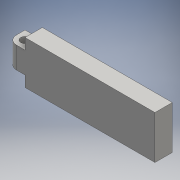
# Autodesk Inventor part: promo3
Saved by Autodesk Inventor 2016 (Build 200138000, 138)
## iProperties
Created: 2016-05-09
Part Number: promo3
Material: 一般
Document SubType Name: Modeling
Designer: 宏太
Density: 1 g/cm^3
Appearance: 既定
Author: 宏太
Autodesk Inventor part; units mm, degrees
ref_plane "YZ Plane" through (0, 0, 0) normal (1, 0, 0) x (0, 1, 0)
ref_plane "XZ Plane" through (0, 0, 0) normal (0, 1, 0) x (-1, 0, 0)
ref_plane "XY Plane" through (0, 0, 0) normal (0, 0, 1) x (1, 0, 0)
sketch "スケッチ1" plane through (0, 0, 0) normal (0, 1, 0) x (-1, 0, 0)
  line L0 (0, 0) -> (30, 0)
  line L1 (30, 10) -> (0, 10)
  line L2 (0, 10) -> (0, 0)
  line L3 (30, 7.5) -> (34, 7.5)
  line L4 (34, 7.5) -> (34, 2.5)
  line L5 (34, 2.5) -> (30, 2.5)
  line L6 (30, 10) -> (30, 7.5)
  line L7 (30, 2.5) -> (30, 0)
  dimension "d0" = 30
  dimension "d1" = 10
  dimension "d5" = 5
  dimension "d6" = 2.5
  constraints: 16 end point, 2 equal length, 2 horizontal, 1 perpendicular, 1 vertical
  measures "d0" distance of L1.end L1.start
  measures "d1" distance of L1.start L0.end
  measures "d5" distance between parallel lines of L3 L5
  measures "d6" distance between parallel lines of L3 L1
extrude "押し出し1" add sketch "スケッチ1" along normal blind 4
sketch "スケッチ2" plane through (0, 0, 0) normal (0, 0, 1) x (1, 0, 0)
  circle A0 centre (-32, 2) radius 1
  line L0 (-34, 4) -> (-30, 4) projected
  line L1 (-34, 0) -> (-34, 4) projected
  point P0 (0, 0)
  dimension "d7" = 2
  dimension "d8" = 2
  dimension "d9" = 2
  constraints: 1 centre point
  measures "d7" diameter of A0
  measures "d8" distance from line of L0 A0.centre
  measures "d9" distance from line of L1 A0.centre
extrude "押し出し2" cut sketch "スケッチ2" along normal blind 10
fillet "フィレット1" radius 2 1 edges at (-34, 0, 5)
